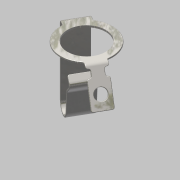
# Autodesk Inventor part: InputJack_signal1
Saved by Autodesk Inventor 2015 SP1 (Build 190203100, 203)
## iProperties
Created: 2015-06-13
Part Number: InputJack_signal1
Material: Generic
Document SubType Name: Modeling
Designer: Peter Mulkers
Density: 1 g/cm^3
Appearance: Titanium
Sheet Metal Rule: Default
Author: Peter Mulkers
Autodesk Inventor part; units mm, degrees
ref_plane "YZ Plane" through (0, 0, 0) normal (1, 0, 0) x (0, 1, 0)
ref_plane "XZ Plane" through (0, 0, 0) normal (0, 1, 0) x (-1, 0, 0)
ref_plane "XY Plane" through (0, 0, 0) normal (0, 0, 1) x (1, 0, 0)
sketch "Sketch1" plane through (0, 0, 0) normal (0, 0, 1) x (1, 0, 0)
  circle A0 centre (0, 0) radius 5.5
  line L0 (-6.928203, 4) -> (6.495191, -3.75) construction
  line L1 (0, 7.5) -> (0, -7.5) construction
  line L2 (-8.553203, 1.185417) -> (-5.303203, 6.814583)
  line L3 (-8.553203, 1.185417) -> (-7.478685, 0.565044)
  line L4 (-5.303203, 6.814583) -> (-4.228685, 6.194209)
  line L5 (7.745191, -1.584936) -> (5.245191, -5.915064)
  line L6 (7.745191, -1.584936) -> (7.373724, -1.37047)
  line L7 (5.245191, -5.915064) -> (4.873724, -5.700597)
  arc A1 (-7.478685, 0.565044) -> (4.873724, -5.700597) centre (0, 0) ccw
  arc A2 (7.373724, -1.37047) -> (-4.228685, 6.194209) centre (0, 0) ccw
  dimension "d0" = 11
  dimension "d2" = 60
  dimension "d3" = 6.5
  dimension "d4" = 8
  dimension "d5" = 15
  dimension "d6" = 5
  dimension "d7" = 7.5
  dimension "d8" = 7.5
  dimension "d9" = 7.5
  dimension "d10" = 2.5
  constraints: 16 end point, 7 point on circle, 4 perpendicular, 3 centre point, 3 midpoint, 2 coincident, 2 parallel, 1 point on line, 1 vertical alignment
  measures "d0" diameter of A0
  measures "d2" angle of L1 L0
  measures "d3" distance of L2.start L2.end
  measures "d4" distance from line of point (0, 0) L2
  measures "d5" distance of L1.start L1.end
  measures "d6" distance of L5.start L5.end
  measures "d7" radius of A2
  measures "d8" radius of A1
  measures "d9" distance from line of L5 A0.centre
  measures "d10" distance between parallel lines of L6 L0
extrude "Extrusion1" add sketch "Sketch1" along normal blind 0.5
sketch "Sketch2" plane through (5.620191, -6.13157, -0.25) normal (0.75, -0.4330127, 0.5) x (0.5, 0.8660254, 0)
  line L0 (5, 0) -> (0, 0)
  line L1 (0, 0) -> (0, -9.42265)
  line L2 (0, -9.42265) -> (5, -9.42265)
  line L3 (5, -9.42265) -> (5, 0)
  constraints: 8 end point
edge flange "Flange1" height 10 angle 60 thickness 0.5 bend radius 0.5 thickness toward (0.75, -0.4330127, 0.5) relief tear relief width 0.5 relief depth 0.25 edges at (6.495191, -3.75, 0) wall of the first edge with corners at (8.120191, -1.801443, -0.25) (5.620191, -6.13157, -0.25) (9.700318, -8.487232, -8.410254) (12.200318, -4.157105, -8.410254)
bend "Bend1"
corner "Corner1"
sketch "Sketch3" plane through (10.075318, -8.703739, -8.160254) normal (0.75, -0.4330127, 0.5) x (0.4330127, -0.25, -0.8660254)
  line L0 (-9.42265, 5) -> (-9.42265, 0) construction
  line L1 (0, 0) -> (-9.42265, 0) construction
  line L2 (0, 5) -> (0, 0) construction
  line L3 (-9.42265, 5) -> (0, 5) construction
  line L4 (-9, 0) -> (-9, 1)
  line L5 (-9, 1) -> (-7, 1)
  line L6 (-7, 1) -> (-7, 0)
  line L7 (-7, 0) -> (-9, 0)
  line L8 (-9, 5) -> (-9, 4)
  line L9 (-9, 4) -> (-7, 4)
  line L10 (-7, 4) -> (-7, 5)
  line L11 (-9, 5) -> (-7, 5)
  point P0 (-13.605662, 2.5)
  dimension "d23" = 1
  dimension "d25" = 2
  dimension "d26" = 7
  dimension "d27" = 1
  dimension "d28" = 2
  dimension "d29" = 7
  constraints: 16 end point, 4 perpendicular, 4 point on line, 2 collinear, 2 vertical
  measures "d23" distance between parallel lines of L5 L1
  measures "d25" distance between parallel lines of L6 L4
  measures "d26" distance between parallel lines of L2 L6
  measures "d27" distance between parallel lines of L3 L9
  measures "d28" distance between parallel lines of L10 L8
  measures "d29" distance between parallel lines of L2 L10
extrude "Extrusion2" cut sketch "Sketch3" against normal blind 0.5
fillet "Fillet1" radius 0.5 10 edges at (6.8567, -6.8455, -2.2231) (5.9907, -6.3455, -0.491) (9.3567, -2.5154, -2.2231) (8.4907, -2.0154, -0.491) (6.4907, -5.4795, -0.491) (7.3567, -5.9795, -2.2231) (8.8567, -3.3814, -2.2231) (7.9907, -2.8814, -0.491) (12.3878, -4.2654, -8.2853) (9.8878, -8.5955, -8.2853)
sketch "Sketch4" plane through (9.760735, -2.748612, -2.531089) normal (0.75, -0.4330127, 0.5) x (0.4330127, -0.25, -0.8660254)
  circle A0 centre (3, -2.5) radius 1.5
  line L0 (6.5, -0.5) -> (6.5, -4.5) projected
  point P0 (-7.105662, -2.5)
  point P1 (6.5, -2.5)
  dimension "d33" = 3
  dimension "d34" = 3.5
  constraints: 1 centre point, 1 horizontal alignment, 1 midpoint
  measures "d33" diameter of A0
  measures "d34" distance from line of A0.centre L0
extrude "Extrusion3" cut sketch "Sketch4" against normal blind 0.5
sketch "Sketch5" plane through (-5.736216, 7.064583, -0.5) normal (-0.8660254, 0.5, 0) x (-0.5, -0.8660254, 0)
  line L0 (6.5, 0) -> (0, 0)
  line L1 (0, 0) -> (0, -19)
  line L2 (0, -19) -> (6.5, -19)
  line L3 (6.5, -19) -> (6.5, 0)
  constraints: 6 end point, 1 horizontal, 1 perpendicular, 1 vertical
edge flange "Flange2" height 20 angle 90 thickness 0.5 bend radius 0.5 thickness toward (-0.8660254, 0.5, 0) relief tear relief width 0.5 relief depth 0.25 edges at (-6.928203, 4, 0) wall of the first edge with corners at (-8.986216, 1.435417, -0.5) (-5.736216, 7.064583, -0.5) (-5.736216, 7.064583, -19.5) (-8.986216, 1.435417, -19.5)
bend "Bend2"
corner "Corner2"
sketch "Sketch6" plane through (-9.419229, 1.685417, -19.5) normal (-0.5, -0.8660254, 0) x (0.8660254, -0.5, 0)
  line L0 (0, 19) -> (0, 0) construction
  arc A0 (0, 0) -> (4.986161, -0.262689) centre (2.5, 0) ccw
  line L1 (16.071068, 20) -> (2.240747, 20)
  line L2 (6, 12.5) -> (6, 6.5) construction
  line L3 (6, 8) -> (7.06066, 9.06066) construction
  line L4 (6, 8) -> (7.06066, 6.93934) construction
  line L5 (7.06066, 6.93934) -> (5.842126, 5.720805)
  line L6 (7.06066, 9.06066) -> (6, 10.12132)
  line L7 (4.986161, -0.262689) -> (5.554768, 5.118774)
  arc A1 (7.06066, 6.93934) -> (7.06066, 9.06066) centre (6, 8) ccw
  arc A2 (5.842126, 5.720805) -> (5.554768, 5.118774) centre (6.549232, 5.013699) ccw
  point P0 (9, 19.5)
  dimension "d47" = 5
  dimension "d48" = 12
  dimension "d50" = 6
  dimension "d51" = 45
  dimension "d52" = 45
  dimension "d53" = 1
  dimension "d54" = 1.5
  dimension "d55" = 1.5
  dimension "d56" = 1.72327
  dimension "d57" = 7.5
  constraints: 13 end point, 6 point on circle, 6 tangent, 3 centre point, 1 point on line, 1 vertical
  measures "d47" diameter of A0
  measures "d48" distance from line of L1 L3.start
  measures "d50" distance from line of L0 L3.start
  measures "d51" angle of L3 L2
  measures "d52" angle of L4 L2
  measures "d53" radius of A2
  measures "d54" radius of A1
  measures "d55" distance of L3.end L6.end
  measures "d56" distance of L4.end L5.end
  measures "d57" distance from line of L2.start L1
contour flange "Contour Flange1" sketch "Sketch6" thickness 0.5 bend radius 0.5 curves A0 L7 A2 L5 A1 L6 edges at (-7.361216, 4.25, -19.5) running between points at (-8.986216, 1.435417, -19.5) (-5.736216, 7.064583, -19.5)
bend "Bend3"
corner "Corner3"
fillet "Corner Round1" radius 0.5 6 edges at (-4.3762, -1.2262, -9.5555) (-1.1262, 4.403, -9.5555) (-7.4787, 0.565, 0.25) (-4.2287, 6.1942, 0.25) (4.8737, -5.7006, 0.25) (7.3737, -1.3705, 0.25)
fillet "Fillet2" radius 0.15 98 edges at (-7.5575, 0.528, 0.5) (-3.4091, -6.6804, 0.5) (4.8878, -5.8074, 0.5) (7.4733, -1.3293, 0.5) (4.0809, 6.2926, 0.5) (-4.236, 6.281, 0.5) (-9.1656, 1.539, 0.2071) (-9.4192, 1.6854, -10) (-7.3681, 0.5012, -21.9965) (-4.8549, -0.9498, -17.072) (-4.529, -1.138, -14.0555) (-3.8322, -1.5403, -13.1699) (-2.924, -2.0646, -11.5) (-3.6107, -1.6681, -10.0858) (-4.0602, -1.2395, -9.4822) (-2.5981, 1.5, -9.3787) (-0.9566, 4.136, -9.4822) (-0.3607, 3.961, -10.0858) (0.326, 3.5646, -11.5) (-0.5822, 4.0889, -13.1699) (-1.279, 4.4912, -14.0555) (-1.6049, 4.6794, -17.072) (-4.1181, 6.1303, -21.9965) (-6.1692, 7.3146, -10) (-5.9156, 7.1681, 0.2071) (8.1489, -1.818, 0.3847) (8.4772, -2.0093, 0.033) (8.5388, -2.245, -0.262) (8.4282, -2.5566, -0.366) (8.3148, -2.8994, -0.4928) (8.6112, -3.2396, -1.2321) (9.2942, -3.0566, -2.0981) (9.054, -3.3262, -1.9713) (9.5344, -2.787, -2.2249) (11.0598, -3.4986, -5.1292) (12.4387, -4.4638, -8.0335) (11.3253, -6.5387, -8.1603) (10.0851, -8.5403, -8.0335) (8.5598, -7.8287, -5.1292) (7.1808, -6.8635, -2.2249) (7.2942, -6.5207, -2.0981) (7.4076, -6.1779, -1.9713) (7.1112, -5.8377, -1.2321) (6.6684, -5.7511, -0.4928) (6.4282, -6.0207, -0.366) (6.2136, -6.2723, -0.262) (5.9787, -6.3368, 0.033) (5.6489, -6.1481, 0.3847) (-4.1383, -1.3635, -12.8164) (-4.9198, -0.9123, -13.8402) (-5.2855, -0.7012, -17.0194) (-7.3453, 0.488, -21.4972) (-8.9862, 1.4354, -10) (-8.8594, 1.3622, -0.1464) (-7.5575, 0.528, 0) (-3.4091, -6.6804, 0) (4.8878, -5.8074, 0) (5.432, -6.0229, -0.0489) (5.6031, -6.12, -0.2173) (5.8386, -6.0558, -0.512) (6.0532, -5.8042, -0.616) (6.2934, -5.5346, -0.7428) (6.7362, -5.6212, -1.4821) (7.0326, -5.9614, -2.2213) (6.9192, -6.3042, -2.3481) (6.8058, -6.647, -2.4749) (8.1848, -7.6122, -5.3792) (9.7101, -8.3238, -8.2835) (10.9503, -6.3222, -8.4103) (12.0637, -4.2473, -8.2835) (10.6848, -3.2821, -5.3792) (8.9192, -2.8401, -2.3481) (9.1594, -2.5705, -2.4749) (8.679, -3.1097, -2.2213) (8.2362, -3.0231, -1.4821) (8.0532, -2.3401, -0.616) (7.9398, -2.6829, -0.7428) (8.1638, -2.0285, -0.512) (8.1016, -1.7924, -0.2173) (7.932, -1.6928, -0.0489) (7.4733, -1.3293, 0) (4.0809, 6.2926, 0) (-4.236, 6.281, 0) (-5.6094, 6.9914, -0.1464) (-5.7362, 7.0646, -10) (-4.0953, 6.1172, -21.4972) (-2.0355, 4.928, -17.0194) (-1.6698, 4.7168, -13.8402) (-0.8883, 4.2657, -12.8164) (-0.1071, 3.8146, -11.5) (-0.6669, 4.1378, -10.4393) (-1.2628, 4.3128, -9.8358) (-2.9043, 1.6768, -9.7322) (-4.3664, -1.0628, -9.8358) (-3.9169, -1.4914, -10.4393) (-3.3571, -1.8146, -11.5) (9.1603, -5.2887, -3.8301) (8.7853, -5.0722, -4.0801)
equation "\"d13\" = BendReliefWidth"
equation "\"d14\" = BendReliefDepth"
equation "\"d15\" = MinimumRemnant"
equation "\"d16\" = BendRadius"
equation "\"d19\" = BendRadius"
equation "\"d20\" = CornerReliefSize"
equation "\"d21\" = GapSize"
equation "\"d22\" = JacobiRadiusSize"
equation "\"d37\" = BendReliefWidth"
equation "\"d38\" = BendReliefDepth"
equation "\"d39\" = MinimumRemnant"
equation "\"d40\" = BendRadius"
equation "\"d43\" = BendRadius"
equation "\"d44\" = CornerReliefSize"
equation "\"d45\" = GapSize"
equation "\"d46\" = JacobiRadiusSize"
equation "\"d59\" = BendReliefWidth"
equation "\"d60\" = BendReliefDepth"
equation "\"d61\" = MinimumRemnant"
equation "\"d62\" = BendRadius"
equation "\"d63\" = BendRadius"
equation "\"d65\" = CornerReliefSize"
equation "\"d66\" = GapSize"
equation "\"d67\" = JacobiRadiusSize"
equation "\"BendRadius\" = Thickness"
equation "\"BendReliefWidth\" = Thickness"
equation "\"BendReliefDepth\" = 0.5 * Thickness"
equation "\"CornerReliefSize\" = 4 * Thickness"
equation "\"MinimumRemnant\" = 2 * Thickness"
equation "\"TransitionRadius\" = BendRadius"
equation "\"JacobiRadiusSize\" = BendRadius"
equation "\"GapSize\" = Thickness"
equation "\"Thickness\" = 0.5"
body "Solid1"
